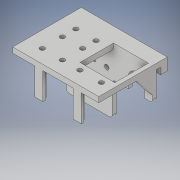
# Autodesk Inventor part: PLACA_BASE
Saved by Autodesk Inventor 2019 (Build 230136000, 136)
## iProperties
Created: 2020-08-25
Part Number: PLACA_BASE
Material: Generic
Document SubType Name: Modeling
Designer: ASUS
Density: 1 g/cm^3
Appearance: Default
Author: ASUS
Autodesk Inventor part; units mm, degrees
ref_plane "YZ Plane" through (0, 0, 0) normal (1, 0, 0) x (0, 1, 0)
ref_plane "XZ Plane" through (0, 0, 0) normal (0, 1, 0) x (-1, 0, 0)
sketch "Sketch1" plane through (0, 0, 0) normal (0, 0, 1) x (1, 0, 0)
  line L0 (0, 0) -> (64, 0)
  line L1 (64, 0) -> (64, 45)
  line L2 (64, 45) -> (0, 45)
  line L3 (0, 45) -> (0, 0)
  circle A0 centre (12, 33) radius 6
  circle A1 centre (52, 33) radius 6
  circle A2 centre (30, 31) radius 1.75
  circle A3 centre (13, 12) radius 1.75
  dimension "d0" = 64
  dimension "d1" = 45
  dimension "d2" = 12
  dimension "d3" = 12
  dimension "d4" = 12
  dimension "d5" = 12
  dimension "d6" = 3.5
  dimension "d7" = 30
  dimension "d8" = 14
  dimension "d9" = 3.5
  dimension "d10" = 13
  dimension "d11" = 33
  constraints: 8 end point, 4 centre point, 2 parallel, 1 equal radius, 1 horizontal, 1 horizontal alignment, 1 perpendicular
  measures "d0" distance of L2.end L1.end
  measures "d1" distance of L1.end L0.end
  measures "d2" distance from line of L3 A0.centre
  measures "d3" distance from line of L1 A1.centre
  measures "d4" distance from line of L2 A0.centre
  measures "d5" diameter of A0
  measures "d6" diameter of A2
  measures "d7" distance from line of L3 A2.centre
  measures "d8" distance from line of L2 A2.centre
  measures "d9" diameter of A3
  measures "d10" distance from line of L3 A3.centre
  measures "d11" distance from line of L2 A3.centre
extrude "Extrusion1" add sketch "Sketch1" along normal blind 3
sketch "Sketch2" plane through (0, 0, 3) normal (0, 0, 1) x (1, 0, 0)
  line L0 (0, 0) -> (64, 0) projected
  line L1 (64, 0) -> (34, 0)
  line L2 (34, 0) -> (34, 25)
  line L3 (34, 25) -> (64, 25)
  line L4 (64, 25) -> (64, 0)
  dimension "d14" = 30
  dimension "d15" = 25
  constraints: 8 end point, 2 parallel, 1 horizontal, 1 perpendicular
  measures "d14" distance of L2.end L3.end
  measures "d15" distance of L1.end L2.end
extrude "Extrusion2" cut sketch "Sketch2" against normal blind 3
fillet "Fillet1" radius 2 4 edges at (34, 25, 1.5) (64, 25, 1.5) (34, 0, 1.5) (0, 0, 1.5)
sketch "Sketch5" plane through (0, 45, 0) normal (0, 1, 0) x (1, 0, 0)
  line L0 (64, -3) -> (0, -3) projected
  line L1 (0, -3) -> (64, -3)
  line L2 (64, -3) -> (64, 8)
  line L3 (64, 8) -> (0, 8)
  line L4 (0, 8) -> (0, -3)
  point P0 (0, 0)
  dimension "d20" = 11
  dimension "d21" = 64
  constraints: 8 end point, 2 parallel, 1 horizontal, 1 perpendicular
  measures "d20" distance of L1.end L2.end
  measures "d21" distance of L2.end L3.end
extrude "Extrusion3" add sketch "Sketch5" along normal blind 4
sketch "Sketch6" plane through (0, 0, 3) normal (0, 0, 1) x (1, 0, 0)
  line L0 (0, 49) -> (64, 49) projected
  line L1 (64, 27) -> (64, 49) projected
  line L2 (0, 49) -> (64, 49)
  line L3 (64, 49) -> (64, 45)
  line L4 (64, 45) -> (0, 45)
  line L5 (0, 45) -> (0, 49)
  point P0 (0, 0)
  dimension "d24" = 4
  constraints: 8 end point, 2 parallel, 1 horizontal, 1 perpendicular, 1 point on line
  measures "d24" distance of L2.end L3.end
extrude "Extrusion4" add sketch "Sketch6" along normal blind 40
sketch "Sketch7" plane through (0, 45, 3) normal (0, -1, 0) x (1, 0, 0)
  line L0 (61, 20) -> (35, 20)
  line L1 (35, 20) -> (35, 0)
  line L2 (35, 0) -> (61, 0)
  line L3 (61, 0) -> (61, 20)
  line L4 (0, 40) -> (64, 40) projected
  line L5 (64, 0) -> (64, 40) projected
  point P0 (0, -3)
  dimension "d27" = 20
  dimension "d28" = 3
  dimension "d29" = 20
  dimension "d30" = 26
  constraints: 8 end point, 2 parallel, 1 horizontal, 1 perpendicular
  measures "d27" distance between parallel lines of L4 L0
  measures "d28" distance between parallel lines of L5 L3
  measures "d29" distance of L2.end L0.start
  measures "d30" distance of L0.start L0.end
extrude "Extrusion5" cut sketch "Sketch7" against normal blind 40
sketch "Sketch8" plane through (0, 45, 43) normal (0, -1, 0) x (1, 0, 0)
  line L0 (35, -20) -> (61, -20) projected
  line L1 (61, -20) -> (61, -40) projected
  line L2 (35, -40) -> (35, -20) projected
  line L3 (35, -40) -> (0, -40) projected
  point P0 (0, -43)
  point P1 (56, -10)
  point P2 (40, -10)
  point P3 (27, -25)
  point P4 (27, -35)
  point P5 (12, -35)
  point P6 (12, -25)
  point P7 (12, -10)
  point P8 (27, -10)
  dimension "d33" = 10
  dimension "d34" = 10
  dimension "d35" = 5
  dimension "d36" = 5
  dimension "d37" = 5
  dimension "d38" = 8
  dimension "d39" = 8
  dimension "d40" = 5
  dimension "d63" = 15
  constraints: 4 horizontal alignment, 3 vertical alignment
  measures "d33" distance from line of L0 point (56, -10)
  measures "d34" distance from line of L0 point (40, -10)
  measures "d35" distance from line of L1 point (56, -10)
  measures "d36" distance from line of L2 point (40, -10)
  measures "d37" distance from line of L0 point (27, -25)
  measures "d38" distance from line of L2 point (27, -25)
  measures "d39" distance from line of L2 point (27, -35)
  measures "d40" distance from line of L3 point (27, -35)
  measures "d63" distance of point (12, -10) point (27, -10)
hole "Hole1" at (56, 45, 33) at (40, 45, 33) at (27, 45, 18) at (27, 45, 8) at (12, 45, 8) at (12, 45, 18) at (12, 45, 33) at (27, 45, 33) direction (0, 1, 0) diameter 3.5 end through all
sketch "Sketch10" plane through (0, 2, 0) normal (-1, 0, 0) x (0, 0, 1)
  line L0 (3, 28) -> (15, 43)
  line L1 (3, 43) -> (43, 43) projected
  line L2 (3, 43) -> (3, 28)
  line L3 (3, 37) -> (3, 25) projected
  line L4 (3, 43) -> (15, 43)
  point P0 (0, -2)
  dimension "d48" = 15
  dimension "d49" = 12
  constraints: 6 end point, 1 collinear, 1 perpendicular, 1 point on line
  measures "d48" distance of L1.start L0.start
  measures "d49" distance of L1.start L0.end
extrude "Extrusion6" add sketch "Sketch10" against normal blind 4
sketch "Sketch11" plane through (64, 27, 3) normal (1, 0, 0) x (0, 0, -1)
  line L0 (0, 0) -> (0, 12) projected
  line L1 (0, 3) -> (0, 18)
  line L2 (0, 18) -> (-12, 18)
  line L3 (0, 18) -> (-20, 18) projected
  line L4 (0, 3) -> (-12, 18)
  point P0 (3, -27)
  dimension "d52" = 12
  dimension "d53" = 15
  constraints: 6 end point, 2 point on line, 1 horizontal, 1 vertical
  measures "d52" distance of L1.end L2.end
  measures "d53" distance of L1.start L1.end
extrude "Extrusion7" add sketch "Sketch11" against normal blind 3
ref_plane "Work Plane1" through (20, 2, 0) normal (-1, 0, 0) x (0, 0, 1)
sketch "Sketch12" plane through (20, 2, 0) normal (-1, 0, 0) x (0, 0, 1)
  line L0 (3, 43) -> (3, 28) projected
  line L1 (3, 43) -> (3, 28)
  line L2 (15, 43) -> (3, 28) projected
  line L3 (3, 28) -> (15, 43)
  line L4 (15, 43) -> (3, 43)
  point P0 (0, -2)
  constraints: 6 end point, 2 collinear, 1 perpendicular
extrude "Extrusion8" add sketch "Sketch12" along normal mid plane 3
sketch "Sketch13" plane through (0, 45, 0) normal (0, -1, 0) x (1, 0, 0)
  line L0 (0, -8) -> (0, 0) projected
  line L1 (64, -8) -> (64, 43) projected
  line L2 (0, -8) -> (64, -8)
  line L3 (64, -8) -> (64, -3)
  line L4 (64, -3) -> (0, -3)
  line L5 (0, -3) -> (0, -8)
  dimension "d59" = 5
  constraints: 8 end point, 2 parallel, 1 horizontal, 1 perpendicular, 1 point on line
  measures "d59" distance of L3.end L2.end
extrude "Extrusion9" add sketch "Sketch13" along normal blind 5
sketch "Sketch14" plane through (0, 45, 43) normal (0, -1, 0) x (1, 0, 0)
  line L0 (64, 0) -> (0, 0) projected
  line L1 (16.5, 0) -> (22.5, 0)
  line L2 (22.5, -2) -> (22.5, 0)
  line L3 (22.5, -2) -> (20.75, -2)
  line L4 (20.75, -2) -> (20.75, -4)
  line L5 (20.75, -4) -> (18.25, -4)
  line L6 (18.25, -4) -> (18.25, -2)
  line L7 (18.25, -2) -> (16.5, -2)
  line L8 (16.5, -2) -> (16.5, 0)
  line L9 (45, 0) -> (45, -2)
  line L10 (45, -2) -> (46.75, -2)
  line L11 (46.75, -2) -> (46.75, -4)
  line L12 (46.75, -4) -> (49.25, -4)
  line L13 (49.25, -4) -> (49.25, -2)
  line L14 (49.25, -2) -> (51, -2)
  line L15 (51, -2) -> (51, 0)
  line L16 (45, 0) -> (51, 0)
  point P0 (0, -43)
  dimension "d64" = 2
  dimension "d65" = 2.5
  dimension "d66" = 6
  dimension "d67" = 2.5
  dimension "d68" = 6
  dimension "d70" = 2
  dimension "d72" = 16.5
  dimension "d73" = 13
  constraints: 32 end point, 12 point on line, 9 perpendicular, 2 collinear, 1 horizontal, 1 parallel
  measures "d64" distance of L9.start L9.end
  measures "d65" distance of L4.end L5.end
  measures "d66" distance between parallel lines of L15 L9
  measures "d67" distance of L11.end L12.end
  measures "d68" distance between parallel lines of L2 L8
  measures "d70" distance of L3.end L4.end
  measures "d72" distance from line of L0.end L8
  measures "d73" distance from line of L0.start L15
extrude "Extrusion10" add sketch "Sketch14" along normal blind 20
sketch "Sketch16" plane through (0, 49, 0) normal (0, 1, 0) x (1, 0, 0)
  line L0 (35, -23) -> (61, -23)
  line L1 (61, -23) -> (61, -28)
  line L2 (61, -28) -> (35, -28)
  line L3 (35, -28) -> (35, -23)
  point P0 (0, 0)
  dimension "d86" = 26
  dimension "d87" = 5
  constraints: 8 end point, 2 parallel, 1 horizontal, 1 perpendicular
  measures "d86" distance of L1.end L2.end
  measures "d87" distance of L0.end L1.end
extrude "Extrusion12" cut sketch "Sketch16" against normal blind 10
sketch "Sketch17" plane through (0, 0, 3) normal (0, 0, 1) x (1, 0, 0)
  circle A0 centre (52, 33) radius 6 projected
  line L0 (62, 25) -> (36, 25) projected
  line L1 (46, 33) -> (58, 33)
  line L2 (58, 33) -> (58, 25)
  line L3 (58, 25) -> (46, 25)
  line L4 (46, 25) -> (46, 33)
  point P0 (0, 0)
  constraints: 8 end point, 2 parallel, 1 coincident, 1 horizontal, 1 horizontal alignment, 1 midpoint, 1 perpendicular, 1 point on line, 1 other
extrude "Extrusion13" cut sketch "Sketch17" against normal blind 10 contours L2 L0 L4 A0 | A0 L1 picked at (51.2908, 31.13)
equation "\"d3\" = d2"
equation "\"d6\" = d9"
equation "\"d34\" = d33"
equation "\"d36\" = d35"
equation "\"d39\" = d38"
equation "\"d40\" = d37"
equation "\"d67\" = d65"
body "Solid1"
